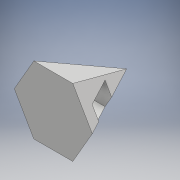
# Autodesk Inventor part: Пирамида
Saved by Autodesk Inventor 2018 (Build 220112000, 112)
## iProperties
Created: 2018-05-16
Part Number: Пирамида
Material: Типовые
Document SubType Name: Modeling
Designer: user
Density: 1 g/cm^3
Appearance: По умолчанию
Author: user
Autodesk Inventor part; units mm, degrees
ref_plane "YZ Plane" through (0, 0, 0) normal (1, 0, 0) x (0, 1, 0)
ref_plane "XZ Plane" through (0, 0, 0) normal (0, 1, 0) x (-1, 0, 0)
ref_plane "XY Plane" through (0, 0, 0) normal (0, 0, 1) x (1, 0, 0)
sketch "Эскиз1" plane through (0, 0, 0) normal (0, 1, 0) x (-1, 0, 0)
  line L0 (42.5, 0) -> (21.25, -36.8061)
  line L1 (21.25, -36.8061) -> (-21.25, -36.8061)
  line L2 (-21.25, -36.8061) -> (-42.5, 0)
  line L3 (-42.5, 0) -> (-21.25, 36.8061)
  line L4 (-21.25, 36.8061) -> (21.25, 36.8061)
  line L5 (21.25, 36.8061) -> (42.5, 0)
  point P0 (0, 0)
  point P1 (0, 0)
  dimension "d0" = 85
  constraints: 12 end point, 1 coincident, 13 other
  measures "d0" distance of L2.end L0.start
sketch "Эскиз2" plane through (0, 0, 0) normal (1, 0, 0) x (0, 1, 0)
  point P0 (0, 0)
  point P1 (80, 0)
  dimension "d1" = 80
  measures "d1" distance of point (0, 0) point (80, 0)
loft "Лофт1" add profiles "Эскиз1" section 2 point at (0, 80, 0)
sketch "Эскиз3" plane through (0, 0, 0) normal (1, 0, 0) x (0, 1, 0)
  line L0 (15, -12.5) -> (45, -12.5)
  line L1 (45, -12.5) -> (45, 12.5)
  line L2 (45, 12.5) -> (15, 12.5)
  line L3 (15, 12.5) -> (15, -12.5)
  line L4 (0, 0) -> (80, 0) projected
  line L5 (15, -12.5) -> (45, 12.5) construction
  line L6 (45, -12.5) -> (15, 12.5) construction
  line L7 (0, 0) -> (0, 36.8061) projected
  point P0 (30, 0)
  dimension "d6" = 30
  dimension "d7" = 25
  dimension "d8" = 15
  constraints: 12 end point, 2 midpoint, 2 parallel, 1 horizontal, 1 perpendicular, 1 point on line
  measures "d6" distance of L2.end L1.end
  measures "d7" distance of L1.end L0.end
  measures "d8" distance from line of L7 L2.end
extrude "Выдавливание1" cut sketch "Эскиз3" along normal through all both and the other way through all
